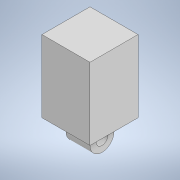
# Autodesk Inventor part: Fallenge
Saved by Autodesk Inventor 2022 (Build 260153000, 153)
## iProperties
Created: 2022-03-12
Part Number: Fallenge
Material: Générique
Document SubType Name: Modeling
Designer: timot
Density: 1 g/cm^3
Appearance: Par défaut
Author: timot
Autodesk Inventor part; units mm, degrees
ref_plane "YZ Plane" through (0, 0, 0) normal (1, 0, 0) x (0, 1, 0)
ref_plane "XZ Plane" through (0, 0, 0) normal (0, 1, 0) x (-1, 0, 0)
ref_plane "XY Plane" through (0, 0, 0) normal (0, 0, 1) x (1, 0, 0)
sketch "Esquisse1" plane through (0, 0, 0) normal (0, 0, 1) x (1, 0, 0)
  line L0 (-10, -15) -> (10, -15)
  line L1 (10, -15) -> (10, 15)
  line L2 (10, 15) -> (-10, 15)
  line L3 (-10, 15) -> (-10, -15)
  line L4 (-10, -15) -> (10, 15) construction
  line L5 (10, -15) -> (-10, 15) construction
  line L6 (-5, -15) -> (-5, -25)
  line L7 (-5, -25) -> (5, -25)
  line L8 (5, -25) -> (5, -15)
  line L9 (0, -15) -> (-5, -25) construction
  line L10 (0, -15) -> (5, -25) construction
  point P0 (0, 0)
  dimension "d0" = 20
  dimension "d1" = 30
  dimension "d4" = 10
  dimension "d5" = 10
  constraints: 22 end point, 3 midpoint, 3 parallel, 2 point on line, 1 horizontal, 1 perpendicular
  measures "d0" distance of L2.end L1.end
  measures "d1" distance of L0.end L1.end
  measures "d4" distance of L6.end L7.end
  measures "d5" distance of L6.start L6.end
extrude "Extrusion1" add sketch "Esquisse1" along normal blind 20
sketch "Esquisse3" plane through (-5, -25, 0) normal (-1, 0, 0) x (0, 0, 1)
  line L0 (5, -10) -> (15, -10)
  line L1 (15, -10) -> (15, 10)
  line L2 (15, 10) -> (5, 10)
  line L3 (5, 10) -> (5, -10)
  line L4 (0, 0) -> (20, 0) projected
  line L5 (5, -10) -> (15, 10) construction
  line L6 (15, -10) -> (5, 10) construction
  line L7 (0, 10) -> (20, 10) projected
  line L8 (5, 0) -> (0, 0)
  line L9 (0, 0) -> (0, 10)
  line L10 (0, 10) -> (5, 10)
  line L11 (5, 10) -> (5, 0)
  line L12 (20, 0) -> (20, 10) projected
  line L13 (15, 0) -> (20, 0)
  line L14 (20, 0) -> (20, 10)
  line L15 (20, 10) -> (15, 10)
  line L16 (15, 10) -> (15, 0)
  point P0 (0, 25)
  point P1 (10, 0)
  dimension "d6" = 10
  constraints: 28 end point, 6 parallel, 5 midpoint, 3 perpendicular, 2 horizontal, 2 point on line
  measures "d6" distance of L0.start L0.end
extrude "Extrusion2" cut sketch "Esquisse3" against normal blind 20 contours L4 L9 L7 L3 | L1 L7 L12 L4
sketch "Esquisse4" plane through (-5, -25, 15) normal (-1, 0, 0) x (0, 0, 1)
  line L0 (-10, 10) -> (-10, 0) projected
  line L1 (-10, 5) -> (0, 5)
  line L2 (0, 0) -> (0, 10) projected
  circle A0 centre (-5, 5) radius 2.5
  point P0 (-15, 25)
  dimension "d9" = 5
  constraints: 3 midpoint, 2 end point, 1 centre point
  measures "d9" diameter of A0
extrude "Extrusion3" cut sketch "Esquisse4" against normal blind 20
fillet "Congé1" radius 5 2 edges at (0, -25, 5) (0, -25, 15)
